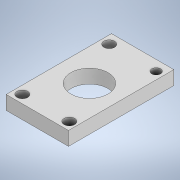
# Autodesk Inventor part: Bloque-Part
Saved by Autodesk Inventor 2020 (Build 240168000, 168)
## iProperties
Created: 2019-10-31
Part Number: Bloque-Part
Material: Generic
Document SubType Name: Modeling
Designer: jsoto
Density: 1 g/cm^3
Appearance: Default
Author: jsoto
Autodesk Inventor part; units mm, degrees
ref_plane "YZ Plane" through (0, 0, 0) normal (1, 0, 0) x (0, 1, 0)
ref_plane "XZ Plane" through (0, 0, 0) normal (0, 1, 0) x (-1, 0, 0)
ref_plane "XY Plane" through (0, 0, 0) normal (0, 0, 1) x (1, 0, 0)
sketch "Sketch2" plane through (0, 0, 0) normal (0, 1, 0) x (-1, 0, 0)
  line L0 (11.5834, 18.5596) -> (-10.9749, 18.5596)
  line L1 (-10.9749, 18.5596) -> (-10.9749, -19.5593)
  line L2 (-10.9749, -19.5593) -> (11.5834, -19.5593)
  line L3 (11.5834, -19.5593) -> (11.5834, 18.5596)
  circle A0 centre (8.6713, 15.6039) radius 1.9409
  circle A1 centre (0, 0) radius 6.7207
  circle A2 centre (-8.3236, 15.6039) radius 1.9409
  circle A3 centre (8.6713, -15.8213) radius 1.9511
  circle A4 centre (-8.3236, -15.8213) radius 1.6029
  constraints: 8 end point, 5 centre point, 2 parallel, 1 coincident, 1 horizontal, 1 perpendicular
extrude "Extrusion2" add sketch "Sketch2" along normal blind 5
body "Solid2"
